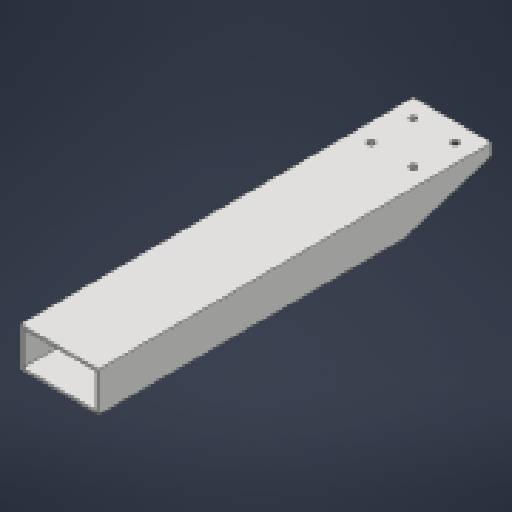
# Autodesk Inventor part: 40x15
Saved by Autodesk Inventor 2025 (Build 290162000, 162)
## iProperties
Created: 2025-04-21
Part Number: 40x15
Material: 常规
Document SubType Name: Modeling
Designer: XH
Density: 1 g/cm^3
Appearance: 默认
Author: XH
Autodesk Inventor part; units mm, degrees
ref_plane "YZ Plane" through (0, 0, 0) normal (1, 0, 0) x (0, 1, 0)
ref_plane "XZ Plane" through (0, 0, 0) normal (0, 1, 0) x (-1, 0, 0)
ref_plane "XY Plane" through (0, 0, 0) normal (0, 0, 1) x (1, 0, 0)
sketch "草图1" plane through (0, 0, 0) normal (0, 0, 1) x (1, 0, 0)
  line L0 (15, -7.5) -> (-15, -7.5)
  line L1 (-15, -7.5) -> (-15, 7.5)
  line L2 (-15, 7.5) -> (15, 7.5)
  line L3 (15, 7.5) -> (15, -7.5)
  line L4 (15, -7.5) -> (-15, 7.5) construction
  line L5 (-15, -7.5) -> (15, 7.5) construction
  line L6 (14, 6.5) -> (-14, 6.5)
  line L7 (-14, 6.5) -> (-14, -6.5)
  line L8 (-14, -6.5) -> (14, -6.5)
  line L9 (14, -6.5) -> (14, 6.5)
  point P0 (0, 0)
  dimension "d0" = 30
  dimension "d1" = 15
  dimension "d2" = 1
  constraints: 20 end point, 4 parallel, 2 midpoint, 2 perpendicular, 1 horizontal, 3 other
  measures "d0" distance of L1.end L2.end
  measures "d1" distance of L0.end L1.end
  measures "d2" distance between parallel lines of L2 L6
extrude "拉伸1" add sketch "草图1" along normal blind 150
sketch "草图2" plane through (-15, -7.5, 0) normal (0, -1, 0) x (1, 0, 0)
  line L0 (-150, 0) -> (30, 0) projected
  line L1 (30, 30) -> (30, 0) projected
  line L2 (-150, 30) -> (30, 30) projected
  line L3 (-150, 30) -> (-150, 0) projected
  circle A0 centre (7, 7) radius 1.35 projected
  circle A1 centre (23, 7) radius 1.35 projected
  circle A2 centre (23, 23) radius 1.35 projected
  circle A3 centre (-109, 7) radius 1.35 projected
  circle A4 centre (7, 23) radius 1.35 projected
  circle A5 centre (-127, 23) radius 1.35 projected
  circle A6 centre (-127, 7) radius 1.35 projected
  circle A7 centre (-143, 7) radius 1.35 projected
  circle A8 centre (-11, 23) radius 1.35 projected
  circle A9 centre (-11, 7) radius 1.35 projected
  circle A10 centre (-109, 23) radius 1.35 projected
  circle A11 centre (-143, 23) radius 1.35 projected
  point P0 (15, 0)
extrude "拉伸2" cut sketch "草图2" against normal blind 23.75 contours A0 | A1 | A2 | A4
sketch "草图3" plane through (-15, -7.5, 0) normal (-1, 0, 0) x (0, 0, 1)
  line L0 (0, 0) -> (0, 15) projected
  line L1 (0, 10.637) -> (33.403, 0)
  line L2 (0, 0) -> (150, 0) projected
  point P0 (0, 7.5)
  constraints: 2 end point, 2 point on line
extrude "拉伸3" cut sketch "草图3" against normal blind 35
